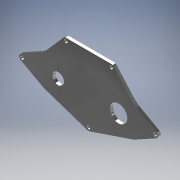
# Autodesk Inventor part: Right Plate
Saved by Autodesk Inventor 2019.4 (Build 234330000, 330)
## iProperties
Created: 2020-01-24
Part Number: Right Plate
Material: Aluminum 6061
Document SubType Name: Modeling
Designer: Mark
Mass: 166.743 g
Surface Area: 295.024 cm^2
Volume: 61.7567 cm^3
Density: 2.7 g/cm^3
Appearance: Aluminum - Flat
Author: Mark
Autodesk Inventor part; units mm, degrees
ref_plane "YZ Plane" through (0, 0, 0) normal (1, 0, 0) x (0, 1, 0)
ref_plane "XZ Plane" through (0, 0, 0) normal (0, 1, 0) x (-1, 0, 0)
ref_plane "XY Plane" through (0, 0, 0) normal (0, 0, 1) x (1, 0, 0)
sketch "Sketch1" plane through (0, 0, 0) normal (0, 0, 1) x (1, 0, 0)
  line L0 (-25, -25) -> (25, -25) construction
  line L1 (25, -25) -> (25, 25) construction
  line L2 (25, 25) -> (-25, 25) construction
  line L3 (-25, 25) -> (-25, -25) construction
  line L4 (-25, -25) -> (25, 25) construction
  line L5 (25, -25) -> (-25, 25) construction
  line L6 (-25, -25) -> (-125, -25) construction
  line L7 (-125, -25) -> (-125, 25) construction
  line L8 (-125, 25) -> (-25, 25) construction
  line L9 (-25, 25) -> (-25, -25) construction
  circle A0 centre (0, 0) radius 14.2875
  circle A1 centre (-12.5, 60) radius 2.75
  circle A2 centre (-87.5, 60) radius 2.75
  circle A3 centre (-160, 0) radius 2.75
  circle A4 centre (60, 0) radius 2.75
  circle A5 centre (-50, -45) radius 2.75
  arc A6 (-9.3122, 63.852) -> (-12.5, 65) centre (-12.5, 60) ccw
  arc A7 (-87.5, 65) -> (-91.2516, 63.3053) centre (-87.5, 60) ccw
  arc A8 (61.8932, -4.6277) -> (62.4135, 4.3789) centre (60, 0) ccw
  arc A9 (-51.8932, -49.6277) -> (-48.1068, -49.6277) centre (-50, -45) ccw
  arc A10 (-163.1878, 3.852) -> (-161.8932, -4.6277) centre (-160, 0) ccw
  line L10 (-12.5, 65) -> (-87.5, 65)
  circle A11 centre (-100, 0) radius 9.5
  line L11 (-163.1878, 3.852) -> (-90.6878, 63.852)
  line L12 (-9.3122, 63.852) -> (63.1878, 3.852)
  line L13 (-161.8932, -4.6277) -> (-51.8932, -49.6277)
  line L14 (-48.1068, -49.6277) -> (61.8932, -4.6277)
  dimension "d1" = 50
  dimension "d2" = 100
  dimension "d3" = 50
  dimension "d4" = 28.575
  dimension "d12" = 5.5
  dimension "d13" = 5.5
  dimension "d14" = 5.5
  dimension "d15" = 5.5
  dimension "d16" = 5.5
  dimension "d17" = 75
  dimension "d18" = 20
  dimension "d19" = 35
  dimension "d20" = 35
  dimension "d21" = 25
  dimension "d23" = 35
  dimension "d24" = 37.5
  dimension "d25" = 25
  dimension "d26" = 37.5
  dimension "d27" = 10
  dimension "d28" = 10
  dimension "d29" = 10
  dimension "d30" = 10
  dimension "d31" = 10
  dimension "d32" = 50
  dimension "d33" = 75
  dimension "d35" = 19
  dimension "d37" = 25
  dimension "d38" = 25
  constraints: 30 end point, 12 centre point, 12 point on circle, 10 tangent, 6 coincident, 4 parallel, 2 horizontal, 2 midpoint, 2 perpendicular
  measures "d1" distance of L1.end L0.end
  measures "d2" distance of L7.end L8.end
  measures "d3" distance of L6.end L7.end
  measures "d4" diameter of A0
  measures "d12" diameter of A1
  measures "d13" diameter of A2
  measures "d14" diameter of A3
  measures "d15" diameter of A4
  measures "d16" diameter of A5
  measures "d17" distance from line of L1 A5.centre
  measures "d18" distance from line of L6 A5.centre
  measures "d19" distance from line of L7 A3.centre
  measures "d20" distance from line of L1 A4.centre
  measures "d21" distance from line of L0 A4.centre
  measures "d23" distance from line of L8 A2.centre
  measures "d24" distance from line of L7 A2.centre
  measures "d25" distance from line of L8 A3.centre
  measures "d26" distance from line of L1 A1.centre
  measures "d27" diameter of A6
  measures "d28" diameter of A7
  measures "d29" diameter of A8
  measures "d30" diameter of A9
  measures "d31" diameter of A10
  measures "d32" distance of L1.end L2.end
  measures "d33" distance of L10.start L10.end
  measures "d35" diameter of A11
  measures "d37" distance from line of L6 A11.centre
  measures "d38" distance from line of L7 A11.centre
extrude "Extrusion1" add sketch "Sketch1" along normal blind 5
body "Solid1"
